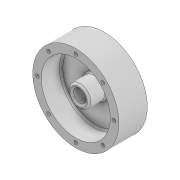
# Autodesk Inventor part: Cycloidal gear cover front
Saved by Autodesk Inventor 2020.3 (Build 243373010, 373A)
## iProperties
Created: 2021-05-02
Part Number: Cycloidal gear cover front
Material: Generic
Document SubType Name: Modeling
Designer: marti
Density: 1 g/cm^3
Appearance: Default
Author: marti
Autodesk Inventor part; units mm, degrees
ref_plane "YZ Plane" through (0, 0, 0) normal (1, 0, 0) x (0, 1, 0)
ref_plane "XZ Plane" through (0, 0, 0) normal (0, 1, 0) x (-1, 0, 0)
ref_plane "XY Plane" through (0, 0, 0) normal (0, 0, 1) x (1, 0, 0)
sketch "Sketch1" plane through (0, 0, 0) normal (0, 0, 1) x (1, 0, 0)
  circle A0 centre (0, 0) radius 50
  point P0 (0, 44.5)
  constraints: 1 centre point
extrude "Extrusion1" add sketch "Sketch1" along normal blind 10
sketch "Sketch4" plane through (0, 0, 10) normal (0, 0, 1) x (1, 0, 0)
  circle A0 centre (0, 0) radius 40
  circle A1 centre (0, 0) radius 50 projected
  dimension "d20" = 80
  constraints: 1 centre point, 1 coincident
  measures "d20" diameter of A0
extrude "Extrusion4" add sketch "Sketch4" along normal blind 23
hole "Hole2" at (0, 44.5, 0) direction (0, 0, 1) diameter 4.134 end through all counterbore diameter 7 counterbore depth 2 thread size "M5x0.8" class "6H" standard "ISO Metric profile"
pattern_circular "Circular Pattern2" count 8 over 360 about axis through (0, 0, -10) along (0, 0, 1) of "Hole2"
sketch "Sketch5" plane through (0, 0, 0) normal (0, 0, -1) x (-1, 0, 0)
  circle A0 centre (0, 0) radius 7.5
  dimension "d34" = 15
  constraints: 1 centre point, 1 coincident
  measures "d34" diameter of A0
extrude "Extrusion5" cut sketch "Sketch5" against normal through all
sketch "Sketch6" plane through (0, 0, 0) normal (0, 0, -1) x (-1, 0, 0)
  circle A0 centre (0, 0) radius 7.5 projected
  circle A1 centre (0, 0) radius 50 projected
sketch "Sketch8" plane through (0, 0, 10) normal (0, 0, 1) x (1, 0, 0)
  circle A0 centre (0, 0) radius 12.5
  circle A1 centre (0, 0) radius 7.5 projected
  dimension "d50" = 25
  constraints: 1 centre point, 1 coincident
  measures "d50" diameter of A0
extrude "Extrusion7" add sketch "Sketch8" along normal blind 20
chamfer "Chamfer1" distance 2 angle 45 2 edges at (-7.5, 0, 30) (-12.5, 0, 30)
fillet "Fillet1" radius 2 2 edges at (-12.5, 0, 10) (-40, 0, 10)
chamfer "Chamfer2" distance 2 angle 45 1 edges at (7.5, 0, 0)
body "Solid1"
